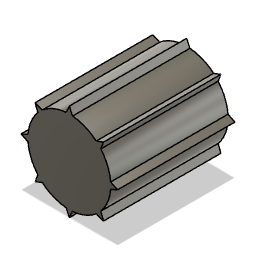
engraneorugas (Autodesk Fusion 360 design; units mm, degrees)
Autodesk Fusion 360 part; units mm, degrees
sketch "Boceto1" plane through (0, 0, 0) normal (0, 0, 1) x (1, 0, 0)
  line L0 (0, 35) -> (-2.3299, 29.9094)
  line L1 (0, 35) -> (2.3299, 29.9094)
  line L2 (-24.7487, 24.7487) -> (-19.5017, 22.7966)
  line L3 (-24.7487, 24.7487) -> (-22.7966, 19.5017)
  line L4 (-35, 0) -> (-29.9094, 2.3299)
  line L5 (-35, 0) -> (-29.9094, -2.3299)
  line L6 (-24.7487, -24.7487) -> (-22.7966, -19.5017)
  line L7 (-24.7487, -24.7487) -> (-19.5017, -22.7966)
  line L8 (0, -35) -> (-2.3299, -29.9094)
  line L9 (0, -35) -> (2.3299, -29.9094)
  line L10 (24.7487, -24.7487) -> (19.5017, -22.7966)
  line L11 (24.7487, -24.7487) -> (22.7966, -19.5017)
  line L12 (35, 0) -> (29.9094, -2.3299)
  line L13 (35, 0) -> (29.9094, 2.3299)
  line L14 (24.7487, 24.7487) -> (22.7966, 19.5017)
  line L15 (24.7487, 24.7487) -> (19.5017, 22.7966)
  arc A0 (-2.3299, 29.9094) -> (-19.5017, 22.7966) centre (0, 0) ccw
  arc A1 (19.5017, 22.7966) -> (2.3299, 29.9094) centre (0, 0) ccw
  arc A2 (29.9094, 2.3299) -> (22.7966, 19.5017) centre (0, 0) ccw
  arc A3 (22.7966, -19.5017) -> (29.9094, -2.3299) centre (0, 0) ccw
  arc A4 (2.3299, -29.9094) -> (19.5017, -22.7966) centre (0, 0) ccw
  arc A5 (-19.5017, -22.7966) -> (-2.3299, -29.9094) centre (0, 0) ccw
  arc A6 (-22.7966, 19.5017) -> (-29.9094, 2.3299) centre (0, 0) ccw
  arc A7 (-29.9094, -2.3299) -> (-22.7966, -19.5017) centre (0, 0) ccw
  dimension "d1" = 60
  dimension "d3" = 360
  constraint coincident A0.centre A1.centre
  constraint coincident L0.end A6
  constraint concentric A0 A6
  constraint concentric A1 A6
  constraint concentric A2 A6
  constraint concentric A3 A6
  constraint concentric A4 A6
  constraint concentric A5 A6
  constraint concentric A6 A7
  measures "d1" diameter of A6
extrude "Extruir1" add sketch "Boceto1" against normal blind 85
